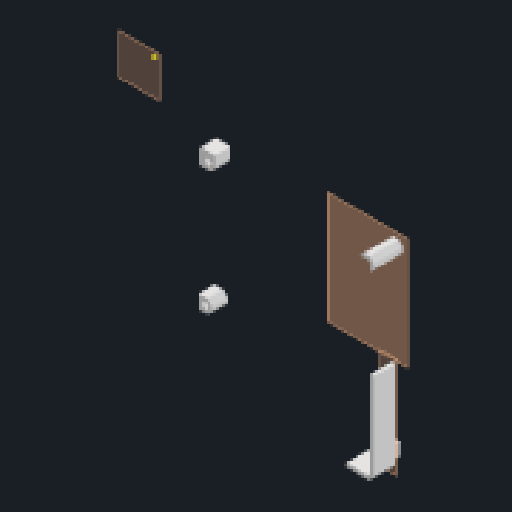
# Autodesk Inventor part: Lid_1
Saved by Autodesk Inventor 2026.2 (Build 302298000, 298)
## iProperties
Created: 2026-04-26
Part Number: Lid_1
Material: Generic
Document SubType Name: Modeling
Designer: Malthe Sennels
Density: 1 g/cm^3
Appearance: Default
Author: Malthe Sennels
Autodesk Inventor part; units mm, degrees
ref_plane "YZ Plane" through (0, 0, 0) normal (1, 0, 0) x (0, 1, 0)
ref_plane "XZ Plane" through (0, 0, 0) normal (0, 1, 0) x (-1, 0, 0)
ref_plane "XY Plane" through (0, 0, 0) normal (0, 0, 1) x (1, 0, 0)
ref_plane "Work Plane1" through (0, 0, 8.4442) normal (0, 0, 1) x (1, 0, 0)
sketch "Sketch1" plane through (0, 0, 8.4442) normal (0, 0, 1) x (1, 0, 0)
  circle A0 centre (126.8952, -26.4793) radius 1.25 projected
  circle A1 centre (37, -26.5) radius 1.25 projected
  circle A2 centre (35.375, -94.25) radius 1.25 projected
  line L0 (132.4, -74.1) -> (132.4, -22.3343) projected
  line L1 (95.5398, -21.1) -> (95.5398, -19.1) projected
  line L2 (131.1657, -21.1) -> (95.5398, -21.1) projected
  line L3 (132.4, -22.3343) -> (131.1657, -21.1) projected
  line L4 (54.6, -116.9) -> (48.6, -116.9) projected
  line L5 (48.6, -116.9) -> (48.6, -121.9) projected
  line L6 (48.6, -121.9) -> (45.5843, -121.9) projected
  line L7 (45.5843, -121.9) -> (31.6, -107.9157) projected
  line L8 (31.6, -107.9157) -> (31.6, -78.9) projected
  line L9 (119.6, -121.9) -> (119.6, -123.9) projected
  line L10 (85.08, -121.9) -> (119.6, -121.9) projected
  line L11 (85.08, -121.9) -> (85.08, -95.9) projected
  line L12 (85.08, -95.9) -> (79.08, -95.9) projected
  line L13 (79.08, -95.9) -> (79.08, -121.9) projected
  line L14 (79.08, -121.9) -> (54.6, -121.9) projected
  line L15 (54.6, -121.9) -> (54.6, -116.9) projected
  circle A3 centre (82.08, -120.16) radius 1.4 projected
  circle A4 centre (51.6, -120.16) radius 1.4 projected
  circle A5 centre (82.08, -98.9) radius 1.4 projected
  line L16 (31.6, -78.9) -> (31.6, -22.3343) projected
  line L17 (31.6, -22.3343) -> (32.8343, -21.1) projected
  line L18 (32.8343, -21.1) -> (40.7204, -21.1) projected
  line L19 (40.7204, -21.1) -> (40.7204, -19.1) projected
  line L20 (126.6, -121.9) -> (126.6, -123.9) projected
  line L21 (126.6, -123.9) -> (131.9941, -123.9) projected
  line L22 (132.4, -74.1) -> (132.4, -120.6657) projected
  line L23 (132.4, -120.6657) -> (131.1657, -121.9) projected
  line L24 (131.1657, -121.9) -> (126.6, -121.9) projected
  line L25 (119.6, -123.9) -> (126.6, -123.9) projected
  line L26 (126.6, -121.9) -> (126.6, -123.9) projected
  line L27 (119.6, -121.9) -> (126.6, -121.9) projected
  line L28 (119.6, -121.9) -> (119.6, -123.9) projected
  circle A6 centre (127.9242, -117.4242) radius 1.25 projected
  line L29 (41.1204, -19.1) -> (41.1204, -21.5)
  line L30 (41.1204, -21.5) -> (33, -21.5)
  line L31 (33, -21.5) -> (32, -22.5)
  line L32 (32, -22.5) -> (32, -78.9)
  line L33 (32, -78.9) -> (32, -107.75)
  line L34 (32, -107.75) -> (45.75, -121.5)
  line L35 (45.75, -121.5) -> (48.2, -121.5)
  line L36 (48.2, -121.5) -> (48.2, -116.5)
  line L37 (48.2, -116.5) -> (55, -116.5)
  line L38 (55, -116.5) -> (55, -121.5)
  line L39 (55, -121.5) -> (78.68, -121.5)
  line L40 (78.68, -121.5) -> (78.68, -95.5)
  line L41 (78.68, -95.5) -> (85.48, -95.5)
  line L42 (85.48, -95.5) -> (85.48, -121.5)
  line L43 (85.48, -121.5) -> (119.6, -121.5)
  line L44 (37, -30.25) -> (31.6, -30.25) projected
  arc A7 (37, -30.25) -> (40.75, -26.5) centre (37, -26.5) ccw projected
  line L45 (40.75, -21.1) -> (40.75, -26.5) projected
  line L46 (123.1452, -26.4793) -> (123.1452, -21.1) projected
  arc A8 (123.1452, -26.4793) -> (126.8952, -30.2293) centre (126.8952, -26.4793) ccw projected
  line L47 (132.4, -30.2293) -> (126.8952, -30.2293) projected
  line L48 (127.9242, -113.6742) -> (132.4, -113.6742) projected
  arc A9 (127.9242, -113.6742) -> (124.1742, -117.4242) centre (127.9242, -117.4242) ccw projected
  line L49 (124.1742, -121.9) -> (124.1742, -117.4242) projected
  line L50 (31.6, -90.5) -> (35.375, -90.5) projected
  arc A10 (35.375, -98) -> (35.375, -90.5) centre (35.375, -94.25) ccw projected
  line L51 (35.375, -98) -> (31.6, -98) projected
  circle A11 centre (37, -26.5) radius 1.75
  circle A12 centre (35.375, -94.25) radius 1.75
  circle A13 centre (127.9242, -117.4242) radius 1.75
  circle A14 centre (126.8952, -26.4793) radius 1.75
  circle A15 centre (126.8952, -26.4793) radius 3.75
  line L52 (129.5469, -29.131) -> (132.4, -26.2779)
  line L53 (124.2436, -23.8277) -> (126.9713, -21.1)
  point P0 (0, 0)
  point P1 (32, -30.25)
  point P2 (40.75, -21.5)
  point P3 (32, -90.5)
  point P4 (32, -98)
  dimension "d0" = 0.4
  dimension "d1" = 3.5
  dimension "d2" = 3.5
  dimension "d3" = 3.5
  dimension "d4" = 3.5
  dimension "d9" = 45
  dimension "d10" = 45
  constraints: 34 end point, 5 centre point, 5 coincident, 2 point on circle, 2 point on line, 2 tangent, 1 concentric, 14 other
  measures "d0" distance between parallel lines of L18 L30
  measures "d1" diameter of A11
  measures "d2" diameter of A12
  measures "d3" diameter of A13
  measures "d4" diameter of A14
  measures "d9" angle of L0 L52
  measures "d10" angle of L2 L53
ref_plane "Work Plane2" through (32, -121.5, 0) normal (0, 0, 1) x (1, 0, 0)
extrude "Extrusion1" add sketch "Sketch1" against normal up to surface (8.4442 mm away) contours L52 A15 L53 L2 L3 L0 | A8 A15 | L32 L31 L30 L45 A7 L44 | L33 L50 A10 L51 | L49 A9 L48 L22 L23 L24 L27
ref_plane "Work Plane3" through (82, -71.5, 4.4442) normal (0, 0, 1) x (1, 0, 0)
sketch "Sketch2" plane through (82, -71.5, 4.4442) normal (0, 0, 1) x (1, 0, 0)
  line L0 (44.6, -50.4) -> (44.6, -52.4) projected
  line L1 (44.6, -52.4) -> (49.9941, -52.4) projected
  line L2 (49.9941, -52.4) -> (52.4, -49.9941) projected
  line L3 (52.4, -49.9941) -> (52.4, -2.6) projected
  line L4 (52.4, -2.6) -> (50.4, -2.6) projected
  line L5 (50.4, -2.6) -> (50.4, -49.1657) projected
  line L6 (50.4, -49.1657) -> (49.1657, -50.4) projected
  line L7 (49.1657, -50.4) -> (44.6, -50.4) projected
  line L8 (37.6, -52.4) -> (44.6, -52.4) projected
  line L9 (44.6, -50.4) -> (44.6, -52.4) projected
  line L10 (37.6, -50.4) -> (44.6, -50.4) projected
  line L11 (37.6, -50.4) -> (37.6, -52.4) projected
  point P0 (-82, 71.5)
extrude "Extrusion2" add sketch "Sketch2" along normal blind 12
ref_plane "Work Plane4" through (116.8408, -46.6, 0.4442) normal (0, 0, 1) x (1, 0, 0)
sketch "Sketch3" plane through (116.8408, -46.6, 0.4442) normal (0, 0, 1) x (1, 0, 0)
  point P0 (-116.8408, 46.6)
ref_plane "Work Plane5" through (116.8408, -46.6, 0.4442) normal (0, 0, 1) x (1, 0, 0)
sketch "Sketch4" plane through (116.8408, -46.6, 0.4442) normal (0, 0, 1) x (1, 0, 0)
  line L0 (15.5592, -27.5) -> (15.5592, 24.2657) projected
  line L1 (17.5592, -27.5) -> (15.5592, -27.5) projected
  line L2 (17.5592, 25.0941) -> (17.5592, -27.5) projected
  line L3 (15.1533, 27.5) -> (17.5592, 25.0941) projected
  line L4 (-21.301, 27.5) -> (15.1533, 27.5) projected
  line L5 (-21.301, 25.5) -> (-21.301, 27.5) projected
  line L6 (14.3249, 25.5) -> (-21.301, 25.5) projected
  line L7 (15.5592, 24.2657) -> (14.3249, 25.5) projected
  line L8 (12.7061, 17.469) -> (15.5592, 20.3221) projected
  line L9 (15.5592, 20.3221) -> (17.5592, 22.3221)
  line L10 (10.1305, 25.5) -> (7.4028, 22.7723) projected
  line L11 (10.1305, 25.5) -> (12.1305, 27.5)
  point P0 (-116.8408, 46.6)
  constraints: 4 end point, 2 collinear, 2 point on line
extrude "Extrusion3" add sketch "Sketch4" along normal up to surface (16 mm away) contours L0 L7 L6 L11 L4 L3 L2 L9
ref_plane "Work Plane6" through (82, -71.5, 4.4442) normal (0, 0, 1) x (1, 0, 0)
sketch "Sketch5" plane through (82, -71.5, 4.4442) normal (0, 0, 1) x (1, 0, 0)
  line L0 (-50.4, -7.4) -> (-52.4, -7.4) projected
  line L1 (-52.4, -7.4) -> (-50.4, -7.4) projected
  line L2 (-50.4, -7.4) -> (-50.4, 49.1657) projected
  line L3 (-50.4, 49.1657) -> (-49.1657, 50.4) projected
  line L4 (-49.1657, 50.4) -> (-41.2796, 50.4) projected
  line L5 (-41.2796, 50.4) -> (-41.2796, 52.4) projected
  line L6 (-41.2796, 52.4) -> (-49.9941, 52.4) projected
  line L7 (-49.9941, 52.4) -> (-52.4, 49.9941) projected
  line L8 (-52.4, 49.9941) -> (-52.4, -7.4) projected
  line L9 (-50.4, -7.2) -> (-52.4, -7.2)
  line L10 (-27.5075, 50.4) -> (-27.5075, 52.4) projected
  line L11 (-27.5075, 52.4) -> (-29.5996, 52.4) projected
  line L12 (-29.5996, 50.4) -> (-29.5996, 52.4) projected
  line L13 (-29.5996, 50.4) -> (-27.5075, 50.4) projected
  line L14 (-10.7816, 50.4) -> (-10.7816, 52.4) projected
  line L15 (-10.7816, 52.4) -> (-12.2675, 52.4) projected
  line L16 (-12.2675, 50.4) -> (-12.2675, 52.4) projected
  line L17 (-12.2675, 50.4) -> (-10.7816, 50.4) projected
  line L18 (-5.7816, 52.4) -> (-5.7816, 50.4) projected
  line L19 (-5.7816, 52.4) -> (-41.2796, 52.4)
  line L20 (-41.2796, 52.4) -> (-41.2796, 50.4)
  line L21 (-41.2796, 50.4) -> (-5.7816, 50.4)
  line L22 (-5.7816, 50.4) -> (-5.7816, 52.4)
  line L23 (-41.2796, 50.4) -> (-50.4, 50.4)
  line L24 (-50.4, 50.4) -> (-50.4, 41.25)
  line L25 (-50.4, 41.25) -> (-41.2796, 41.25)
  line L26 (-41.2796, 41.25) -> (-41.2796, 50.4)
  arc A0 (-45, 41.25) -> (-41.25, 45) centre (-45, 45) ccw projected
  circle A1 centre (-45, 45) radius 1.75 projected
  point P0 (-82, 71.5)
  point P1 (-51.4, -7.2)
  point P2 (-50, 41.25)
  point P3 (-41.2796, 44.5297)
  dimension "d13" = 0.2
  constraints: 18 end point, 4 parallel, 4 point on line, 3 perpendicular, 2 horizontal, 1 midpoint
  measures "d13" distance from line of L0 point (-51.4, -7.2)
extrude "Extrusion4" add sketch "Sketch5" along normal up to surface (12 mm away) contours L9 L8 L7 L6 L5 L4 L23 L24 L2 | L2 L3 L4 L26 A0 L25 | L24 L23 L3 | L19 L12 L21 L5 | L11 L10 L13 L12 | L19 L16 L21 L10 | L15 L14 L17 L16 | L19 L18 L21 L14
sketch "Sketch6" plane through (124.1742, -121.9, 8.4442) normal (0, 1, 0) x (1, 0, 0)
  line L0 (-4.5742, -3) -> (2.4258, 4) projected
  line L1 (-4.5742, 4) -> (-4.5742, -8) projected
  line L2 (0, 4) -> (-4.5742, 4) projected
  line L3 (-4.4328, -3.1414) -> (2.5672, 3.8586)
  line L4 (-4.2913, -3) -> (-4.5742, -3.2828)
  line L5 (2.5672, 3.8586) -> (2.7087, 4)
  line L6 (6.9915, 4) -> (0, 4) projected
  point P0 (-124.1742, 8.4442)
  point P1 (-4.4328, -3.1414)
  dimension "d16" = 0.2
  constraints: 6 end point, 3 point on line, 1 parallel
  measures "d16" distance between parallel lines of L0 L3
extrude "Extrusion5" cut sketch "Sketch6" against normal blind 10
sketch "Sketch7" plane through (128.9713, -19.1, 0.4442) normal (0, 1, 0) x (1, 0, 0)
  arc A0 (-33.4314, 0) -> (-44.8319, -9) centre (-37.9713, -5.9699) ccw projected
  line L0 (-52.7529, -9) -> (-44.8319, -9) projected
  line L1 (0, 0) -> (0, -16) projected
  line L2 (-52.7529, -9) -> (0, -9)
  line L3 (0, -9) -> (0, -16)
  line L4 (0, -16) -> (-52.7529, -16)
  line L5 (-52.7529, -16) -> (-52.7529, -9)
  circle A1 centre (-37.9713, -5.9699) radius 7.5
  line L6 (5.4287, -4) -> (3.4287, -4) projected
  line L7 (3.4287, -4) -> (-52.7529, -4)
  line L8 (-52.7529, -4) -> (-52.7529, -16)
  line L9 (-52.7529, -16) -> (3.4287, -16)
  line L10 (3.4287, -16) -> (3.4287, -4)
  line L11 (3.0228, 0) -> (3.0228, -16) projected
  point P0 (-128.9713, 0.4442)
  point P1 (-31.1106, -9)
  point P2 (-45.2079, -4)
  point P3 (0, -4)
  point P4 (-30.7346, -4)
  constraints: 16 end point, 4 parallel, 2 horizontal, 2 perpendicular, 1 coincident, 3 other
extrude "Extrusion6" add sketch "Sketch7" against normal up to surface (2 mm away) contours L7 L1 L2 A1 | A1 L2 L1 L4 L5 L0
sketch "Sketch8" plane through (128.9713, -19.1, 0.4442) normal (0, 1, 0) x (1, 0, 0)
  line L0 (-57.7529, -4) -> (-52.7529, -9) projected
  line L1 (-52.7529, -4) -> (-52.7529, -9) projected
  line L2 (-52.7529, -4) -> (-96.9654, -4) projected
  point P0 (-128.9713, 0.4442)
extrude "Extrusion7" cut sketch "Sketch8" against normal up to surface (2 mm away)
sketch "Sketch9" plane through (134.4, -121.4941, 4.4442) normal (1, 0, 0) x (0, 0, -1)
  line L0 (0, 47.3941) -> (-12, 47.3941) projected
  line L1 (4, 97.2162) -> (-12, 97.2162) projected
  line L2 (-12, 47.3941) -> (0, 47.3941)
  line L3 (0, 47.3941) -> (0, 97.2162)
  line L4 (0, 97.2162) -> (-12, 97.2162)
  line L5 (-12, 97.2162) -> (-12, 47.3941)
  point P0 (4.4442, 121.4941)
  constraints: 8 end point, 2 parallel, 2 point on line, 1 horizontal, 1 perpendicular
extrude "Extrusion8" add sketch "Sketch9" against normal up to surface (2 mm away)
ref_plane "Work Plane7" through (62.1, -101.4, 11.4442) normal (0, 0, 1) x (1, 0, 0)
sketch "Sketch10" plane through (62.1, -101.4, 11.4442) normal (0, 0, 1) x (1, 0, 0)
  line L0 (-7.5, -15.5) -> (-13.5, -15.5) projected
  line L1 (-13.5, -15.5) -> (-13.5, -20.5) projected
  line L2 (-13.5, -20.5) -> (-16.5157, -20.5) projected
  line L3 (-16.5157, -20.5) -> (-30.5, -6.5157) projected
  line L4 (-30.5, -6.5157) -> (-30.5, 22.5) projected
  line L5 (-30.5, 22.5) -> (-32.5, 22.5) projected
  line L6 (-32.5, 22.5) -> (-32.5, -20.0941) projected
  line L7 (-32.5, -20.0941) -> (-30.0941, -22.5) projected
  line L8 (-30.0941, -22.5) -> (57.5, -22.5) projected
  line L9 (57.5, -20.5) -> (57.5, -22.5) projected
  line L10 (22.98, -20.5) -> (57.5, -20.5) projected
  line L11 (22.98, -20.5) -> (22.98, 5.5) projected
  line L12 (22.98, 5.5) -> (16.98, 5.5) projected
  line L13 (16.98, 5.5) -> (16.98, -20.5) projected
  line L14 (16.98, -20.5) -> (-7.5, -20.5) projected
  line L15 (-7.5, -20.5) -> (-7.5, -15.5) projected
  circle A0 centre (19.98, -18.76) radius 1.4 projected
  circle A1 centre (-10.5, -18.76) radius 1.4 projected
  circle A2 centre (19.98, 2.5) radius 1.4 projected
  line L16 (57.5, -20.5) -> (22.98, -20.5)
  line L17 (22.98, -20.5) -> (22.98, -22.5)
  line L18 (22.98, -22.5) -> (57.5, -22.5)
  line L19 (57.5, -22.5) -> (57.5, -20.5)
  line L20 (-32.5, 22.7) -> (-30.5, 22.7) projected
  line L21 (-32.5, 22.7) -> (-30.5, 22.7)
  line L22 (-30.5, 22.7) -> (-30.5, -6.5157)
  line L23 (-30.5, -6.5157) -> (-32.5, -6.5157)
  line L24 (-32.5, -6.5157) -> (-32.5, 22.7)
  line L25 (-13.5, -20.5) -> (22.98, -20.5)
  line L26 (22.98, -20.5) -> (22.98, -22.5)
  line L27 (22.98, -22.5) -> (-13.5, -22.5)
  line L28 (-13.5, -22.5) -> (-13.5, -20.5)
  point P0 (-62.1, 101.4)
  constraints: 24 end point, 6 parallel, 3 horizontal, 3 perpendicular, 1 point on line
extrude "Extrusion9" add sketch "Sketch10" along normal up to surface (5 mm away) contours L28 L8 L7 L6 L23 L3 L2 | L10 L9 L8 L17 | L23 L6 L5 L4 | L5 L24 L20 L22
sketch "Sketch11" plane through (82, -71.5, 16.4442) normal (0, 0, 1) x (1, 0, 0)
  line L0 (-49.9941, -52.4) -> (-52.4, -49.9941) projected
  line L1 (-33.4, -52.4) -> (-49.9941, -52.4) projected
  line L2 (-52.4, -49.9941) -> (-52.4, 49.9941) projected
  line L3 (-52.4, 49.9941) -> (-49.9941, 52.4) projected
  line L4 (-49.9941, 52.4) -> (49.9941, 52.4) projected
  line L5 (49.9941, 52.4) -> (52.4, 49.9941) projected
  line L6 (52.4, -49.9941) -> (52.4, 49.9941) projected
  line L7 (49.9941, -52.4) -> (52.4, -49.9941) projected
  line L8 (49.9941, -52.4) -> (3.08, -52.4) projected
  line L9 (3.08, -50.4) -> (49.1657, -50.4)
  line L10 (49.1657, -50.4) -> (50.4, -49.1657)
  line L11 (50.4, -49.1657) -> (50.4, 49.1657)
  line L12 (50.4, 49.1657) -> (49.1657, 50.4)
  line L13 (49.1657, 50.4) -> (-49.1657, 50.4)
  line L14 (-49.1657, 50.4) -> (-50.4, 49.1657)
  line L15 (-50.4, 49.1657) -> (-50.4, -49.1657)
  line L16 (-50.4, -49.1657) -> (-49.1657, -50.4)
  line L17 (-49.1657, -50.4) -> (-33.4, -50.4)
  line L18 (3.08, -50.4) -> (-33.4, -50.4)
  point P0 (-82, 71.5)
  dimension "d27" = 2
  constraints: 20 end point, 1 collinear, 8 other
  measures "d27" distance between parallel lines of L8 L9
extrude "Extrusion10" cut sketch "Sketch11" against normal blind 3
sketch "Sketch12" plane through (0, 0, 8.4442) normal (0, 0, 1) x (1, 0, 0)
  line L0 (35.375, -90.5) -> (32, -90.5) projected
  line L1 (32, -90.5) -> (32, -98) projected
  line L2 (32, -98) -> (35.375, -98) projected
  arc A0 (35.375, -98) -> (35.375, -90.5) centre (35.375, -94.25) ccw projected
  circle A1 centre (35.375, -94.25) radius 1.75 projected
  line L3 (39.1, -90.75) -> (31.6, -90.75) projected
  line L4 (31.6, -90.75) -> (31.6, -120.6657) projected
  line L5 (31.6, -120.6657) -> (32.8343, -121.9) projected
  line L6 (32.8343, -121.9) -> (48.6, -121.9) projected
  line L7 (48.6, -121.9) -> (48.6, -117.0555) projected
  line L8 (48.6, -95.9) -> (85.08, -95.9) projected
  line L9 (85.08, -95.9) -> (85.08, -121.9) projected
  line L10 (85.08, -121.9) -> (131.1657, -121.9) projected
  line L11 (131.1657, -121.9) -> (132.4, -120.6657) projected
  line L12 (132.4, -120.6657) -> (132.4, -22.3343) projected
  line L13 (132.4, -22.3343) -> (131.1657, -21.1) projected
  line L14 (131.1657, -21.1) -> (32.8343, -21.1) projected
  line L15 (32.8343, -21.1) -> (31.6, -22.3343) projected
  line L16 (31.6, -22.3343) -> (31.6, -43.25) projected
  line L17 (31.6, -43.25) -> (39.1, -43.25) projected
  line L18 (39.1, -43.25) -> (39.1, -90.75) projected
  circle A2 centre (127.9242, -117.4242) radius 1.75 projected
  circle A3 centre (126.8952, -26.4793) radius 1.75 projected
  line L19 (39.1, -90.75) -> (31.6, -90.75) projected
  line L20 (31.6, -90.75) -> (31.6, -120.6657) projected
  line L21 (31.6, -120.6657) -> (32.8343, -121.9) projected
  line L22 (32.8343, -121.9) -> (48.6, -121.9) projected
  line L23 (48.6, -121.9) -> (48.6, -117.0555) projected
  line L24 (48.6, -95.9) -> (85.08, -95.9) projected
  line L25 (85.08, -95.9) -> (85.08, -121.9) projected
  line L26 (85.08, -121.9) -> (131.1657, -121.9) projected
  line L27 (131.1657, -121.9) -> (132.4, -120.6657) projected
  line L28 (132.4, -120.6657) -> (132.4, -22.3343) projected
  line L29 (132.4, -22.3343) -> (131.1657, -21.1) projected
  line L30 (131.1657, -21.1) -> (32.8343, -21.1) projected
  line L31 (32.8343, -21.1) -> (31.6, -22.3343) projected
  line L32 (31.6, -22.3343) -> (31.6, -43.25) projected
  line L33 (31.6, -43.25) -> (39.1, -43.25) projected
  line L34 (39.1, -43.25) -> (39.1, -90.75) projected
  circle A4 centre (127.9242, -117.4242) radius 1.75 projected
  circle A5 centre (126.8952, -26.4793) radius 1.75 projected
  arc A6 (124.2436, -23.8277) -> (129.5469, -29.131) centre (126.8952, -26.4793) ccw projected
  line L35 (129.5469, -29.131) -> (132.4, -26.2779) projected
  line L36 (126.9713, -21.1) -> (124.2436, -23.8277) projected
  line L37 (124.1742, -117.4242) -> (124.1742, -121.9) projected
  arc A7 (127.9242, -113.6742) -> (124.1742, -117.4242) centre (127.9242, -117.4242) ccw projected
  line L38 (132.4, -113.6742) -> (127.9242, -113.6742) projected
  line L39 (124.1742, -121.9) -> (131.1657, -121.9) projected
  line L40 (131.1657, -121.9) -> (132.4, -120.6657) projected
  line L41 (132.4, -120.6657) -> (132.4, -113.6742) projected
  line L42 (47.8517, -103.0555) -> (48.6, -103.0555) projected
  line L43 (48.6, -103.0555) -> (48.6, -95.9) projected
  line L44 (48.6, -117.0555) -> (47.8517, -117.0555) projected
  line L45 (47.8517, -117.0555) -> (47.8517, -103.0555) projected
  line L46 (47.8517, -103.0555) -> (48.6, -103.0555) projected
  line L47 (48.6, -103.0555) -> (48.6, -95.9) projected
  line L48 (48.6, -117.0555) -> (47.8517, -117.0555) projected
  line L49 (47.8517, -117.0555) -> (47.8517, -103.0555) projected
  point P0 (0, 0)
ref_plane "Work Plane8" through (31.6, -121.9, 13.4442) normal (0, 0, -1) x (0, 1, 0)
extrude "Extrusion11" add sketch "Sketch12" along normal up to surface (5 mm away) contours A0 L3 L1 L0 | A0 L2 L1 L3 | L14 L13 L12 L35 A6 L36 | L12 L11 L10 L37 A7 L38
sketch "Sketch13" plane through (32, -98, 13.4442) normal (0, 0, 1) x (1, 0, 0)
  line L0 (8.6884, -3.1598) -> (-0.4, -3.1598)
  line L1 (-0.4, -3.1598) -> (-0.4, 9.3466)
  line L2 (-0.4, 9.3466) -> (8.6884, 9.3466)
  line L3 (8.6884, 9.3466) -> (8.6884, -3.1598)
  line L4 (-0.4, -22.6657) -> (-0.4, 75.6657) projected
  point P0 (-32, 98)
  constraints: 8 end point, 2 parallel, 1 horizontal, 1 perpendicular, 1 point on line
extrude "Extrusion12" cut sketch "Sketch13" against normal up to surface (13.4442 mm away)
body "Solid1"
